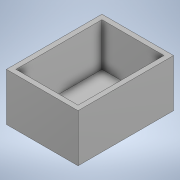
# Autodesk Inventor part: Battery Bucket
Saved by Autodesk Inventor 2022 (Build 260153000, 153)
## iProperties
Created: 2021-12-06
Part Number: Battery Bucket
Material: Generic
Document SubType Name: Modeling
Designer: Vedic
Density: 1 g/cm^3
Appearance: Default
Author: Vedic
Autodesk Inventor part; units mm, degrees
ref_plane "YZ Plane" through (0, 0, 0) normal (1, 0, 0) x (0, 1, 0)
ref_plane "XZ Plane" through (0, 0, 0) normal (0, 1, 0) x (-1, 0, 0)
ref_plane "XY Plane" through (0, 0, 0) normal (0, 0, 1) x (1, 0, 0)
sketch "Sketch1" plane through (0, 0, 0) normal (0, 1, 0) x (-1, 0, 0)
  line L0 (161.2049, 265.4562) -> (-219.7951, 265.4562)
  line L1 (-219.7951, 265.4562) -> (-219.7951, -242.5438)
  line L2 (-219.7951, -242.5438) -> (161.2049, -242.5438)
  line L3 (161.2049, -242.5438) -> (161.2049, 265.4562)
  point P0 (0, 0)
  dimension "d0" = 508
  dimension "d1" = 381
  constraints: 8 end point, 2 parallel, 1 horizontal, 1 perpendicular
  measures "d0" distance of L2.end L0.start
  measures "d1" distance of L1.end L2.end
extrude "Extrusion1" add sketch "Sketch1" along normal blind 25.4
sketch "Sketch2" plane through (0, 25.4, 0) normal (0, 1, 0) x (1, 0, 0)
  line L0 (-161.2049, -265.4562) -> (219.7951, -265.4562) projected
  line L1 (219.7951, -265.4562) -> (-161.2049, -265.4562)
  line L2 (-161.2049, 242.5438) -> (-161.2049, -265.4562) projected
  line L3 (-161.2049, -265.4562) -> (-161.2049, 242.5438)
  line L4 (219.7951, -265.4562) -> (219.7951, 242.5438) projected
  line L5 (-161.2049, 242.5438) -> (219.7951, 242.5438)
  line L6 (219.7951, 242.5438) -> (219.7951, -265.4562)
  line L7 (219.7951, -265.4562) -> (-161.2049, -265.4562)
  line L8 (219.7951, 242.5438) -> (-161.2049, 242.5438) projected
  line L9 (-161.2049, 242.5438) -> (219.7951, 242.5438)
  line L10 (-135.8049, -240.0562) -> (194.3951, -240.0562)
  line L11 (194.3951, -240.0562) -> (194.3951, 217.1438)
  line L12 (194.3951, 217.1438) -> (-135.8049, 217.1438)
  line L13 (-135.8049, 217.1438) -> (-135.8049, -240.0562)
  point P0 (0, 0)
  dimension "d4" = 25.4
  constraints: 20 end point, 4 perpendicular, 2 horizontal, 3 other
  measures "d4" distance between parallel lines of L2 L13
extrude "Extrusion2" add sketch "Sketch2" along normal blind 228.6
sketch "Sketch4" plane through (0, 0, 0) normal (0, -1, 0) x (1, 0, 0)
  line L0 (-161.2049, 265.4562) -> (219.7951, 265.4562) construction
  line L1 (70.5701, 265.4562) -> (70.5701, -242.5438) construction
  line L2 (219.7951, -242.5438) -> (-161.2049, -242.5438) construction
  line L3 (219.7951, 265.4562) -> (219.7951, -242.5438) construction
  circle A0 centre (70.5701, 126.8865) radius 6.35
  circle A1 centre (70.5701, -103.9741) radius 6.35
  line L4 (-161.2049, -242.5438) -> (-161.2049, 265.4562) construction
  line L5 (-161.2049, 11.4562) -> (219.7951, 11.4562) construction
  point P0 (0, 0)
  dimension "d8" = 149.225
  dimension "d9" = 12.7
  dimension "d14" = 138.5697
  dimension "d15" = 138.5697
  constraints: 4 end point, 4 point on line, 2 centre point, 2 midpoint, 1 equal radius, 1 vertical
  measures "d8" distance between parallel lines of L3 L1
  measures "d9" diameter of A0
  measures "d14" distance from line of L2 A1.centre
  measures "d15" distance from line of L0 A0.centre
extrude "Extrusion3" cut sketch "Sketch4" against normal through all
equation "\"d14\" = d11"
equation "\"d11\" = d10"
equation "\"d10\" = 138.5697"
body "Solid1"
